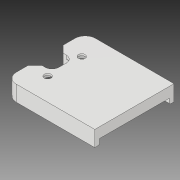
# Autodesk Inventor part: Kondensatorschutz
Saved by Autodesk Inventor 2019.4 (Build 234330000, 330)
## iProperties
Part Number: Kondensatorschutz
Material: PC/ABS-Kunststoff
Document SubType Name: Modeling
Designer: rYan
Density: 0.357273 g/cm^3
Appearance: Glatt - Weiß
Mass: 0.598763 g
Surface Area: 16.4713 cm^2
Volume: 1.67593 cm^3
Author: rYan
Autodesk Inventor part; units mm, degrees
ref_plane "YZ Plane" through (0, 0, 0) normal (1, 0, 0) x (0, 1, 0)
ref_plane "XZ Plane" through (0, 0, 0) normal (0, 1, 0) x (-1, 0, 0)
ref_plane "XY Plane" through (0, 0, 0) normal (0, 0, 1) x (1, 0, 0)
sketch "Skizze1" plane through (0, 0, 0) normal (0, 0, 1) x (1, 0, 0)
  line L0 (3, 11.6) -> (26, 11.6)
  line L1 (26, 11.6) -> (26, -11.6)
  line L2 (26, -11.6) -> (3, -11.6)
  line L3 (0, -8.6) -> (0, 8.6)
  line L4 (-5.9456, 0) -> (31.3243, 0) projected
  arc A0 (3, 11.6) -> (0, 8.6) centre (3, 8.6) ccw
  arc A1 (0, -8.6) -> (3, -11.6) centre (3, -8.6) ccw
  point P0 (0, 0)
  point P1 (0, 11.6)
  dimension "d0" = 23.2
  dimension "d1" = 26
  dimension "d2" = 3
  constraints: 8 end point, 4 point on circle, 4 tangent, 2 centre point, 2 parallel, 2 point on line, 1 equal radius, 1 horizontal, 1 midpoint, 1 perpendicular, 1 other
  measures "d0" distance of L0.end L1.end
  measures "d1" distance of point (0, 11.6) L0.end
  measures "d2" radius of A0
extrude "Extrusion1" add sketch "Skizze1" along normal blind 3
sketch "Skizze2" plane through (0, 0, 0) normal (0, 0, -1) x (-1, 0, 0)
  line L0 (0, -8.6) -> (0, 8.6) projected
  arc A0 (0, 8.6) -> (-3, 11.6) centre (-3, 8.6) ccw projected
  line L1 (-3, 11.6) -> (-26, 11.6) projected
  line L2 (-26, 11.6) -> (-26, -11.6) projected
  line L3 (-26, -11.6) -> (-3, -11.6) projected
  arc A1 (-3, -11.6) -> (0, -8.6) centre (-3, -8.6) ccw projected
  line L4 (-3, -10.2) -> (-26, -10.2)
  line L5 (-26, -10.2) -> (-26, 10.2)
  line L6 (-26, 10.2) -> (-3, 10.2)
  arc A2 (-1.4, 8.6) -> (-3, 10.2) centre (-3, 8.6) ccw
  line L7 (-1.4, 8.6) -> (-1.4, -8.6)
  arc A3 (-3, -10.2) -> (-1.4, -8.6) centre (-3, -8.6) ccw
  line L8 (0, -8.6) -> (0, 8.6) projected
  point P0 (0, 0)
  dimension "d8" = 1.4
  constraints: 8 end point, 4 point on circle, 2 centre point, 1 collinear, 1 tangent, 3 other
  measures "d8" distance between parallel lines of L3 L4
extrude "Extrusion2" add sketch "Skizze2" along normal blind 1.6 contours A1 L3 L2 L4 A3 L7 A2 L6 L1 A0 L0
sketch "Skizze3" plane through (0, 0, 3) normal (0, 0, 1) x (1, 0, 0)
  line L0 (0, 8.6) -> (0, -8.6) projected
  arc A0 (0, -8.6) -> (3, -11.6) centre (3, -8.6) ccw projected
  line L1 (3, -11.6) -> (26, -11.6) projected
  line L2 (26, -11.6) -> (26, 11.6) projected
  line L3 (26, 11.6) -> (3, 11.6) projected
  arc A1 (3, 11.6) -> (0, 8.6) centre (3, 8.6) ccw projected
  line L4 (0, 8.6) -> (0, -8.6) projected
  line L5 (0, 3.1) -> (5, 3.1)
  line L6 (5, 3.1) -> (5, -3.1)
  line L7 (5, -3.1) -> (0, -3.1)
  line L8 (0, -3.1) -> (0, 3.1)
  line L9 (-5.6971, 0) -> (31.2828, 0) projected
  point P0 (0, 0)
  dimension "d9" = 8.5
  dimension "d10" = 5
  constraints: 8 end point, 2 parallel, 1 horizontal, 1 perpendicular, 1 point on line, 1 other
  measures "d9" distance between parallel lines of L3 L5
  measures "d10" distance of L5.start L5.end
extrude "Extrusion3" cut sketch "Skizze3" against normal through all contours L5 L6 L9 L0 | L9 L6 L7 L0
sketch "Skizze5" plane through (0, 0, 0) normal (0, 0, -1) x (-1, 0, 0)
  line L0 (-5, -3.1) -> (-5, 3.1) projected
  line L1 (-31.2, 0) -> (5.2, 0) projected
  line L2 (-5, 3.1) -> (-5, -3.1) projected
  line L3 (-5, -3.1) -> (-9.4, -3.1)
  line L4 (-9.4, -3.1) -> (-9.4, 3.1)
  line L5 (-9.4, 3.1) -> (-5, 3.1)
  line L6 (-5, 3.1) -> (-5, -3.1)
  line L7 (-1.4, -8.6) -> (-1.4, -3.1) projected
  point P0 (0, 0)
  dimension "d23" = 8
  constraints: 8 end point, 2 parallel, 1 horizontal, 1 perpendicular, 1 point on line
  measures "d23" distance between parallel lines of L4 L7
extrude "Extrusion4" cut sketch "Skizze5" against normal blind 2
sketch "Skizze4" plane through (0, 0, 0) normal (0, 0, -1) x (-1, 0, 0)
  line L0 (0, -16.24) -> (0, 16.24) projected
  line L1 (-31.2, 0) -> (5.2, 0) projected
  line L2 (-1.4, -3.1) -> (-1.4, -8.6) projected
  point P0 (0, 0)
  point P1 (-5.6, -5)
  point P2 (-5.6, 5)
  dimension "d13" = 10
  dimension "d15" = 4.2
  constraints: 1 symmetric about line
  measures "d13" distance of point (-5.6, 5) point (-5.6, -5)
  measures "d15" distance from line of point (-5.6, -5) L2
hole "Bohrung1" at (5.6, -5, 0) at (5.6, 5, 0) direction (0, 0, 1) diameter 2 end through all countersink diameter 7 countersink angle 90
fillet "Rundung1" radius 2 2 edges at (5, 3.1, 2.5) (5, -3.1, 2.5)
sketch "Skizze6" plane through (0, 0, -1.6) normal (0, 0, -1) x (-1, 0, 0)
  line L0 (0, -3.1) -> (-1.4, -3.1) projected
  line L1 (-1.4, -3.1) -> (-1.4, -8.6) projected
  arc A0 (-3, -10.2) -> (-1.4, -8.6) centre (-3, -8.6) ccw projected
  line L2 (-3, -10.2) -> (-26, -10.2) projected
  line L3 (-26, -10.2) -> (-26, -11.6) projected
  line L4 (-26, -11.6) -> (-3, -11.6) projected
  arc A1 (-3, -11.6) -> (0, -8.6) centre (-3, -8.6) ccw projected
  line L5 (0, -8.6) -> (0, -3.1) projected
  line L6 (-1.4, 3.1) -> (0, 3.1) projected
  line L7 (0, 3.1) -> (0, 8.6) projected
  arc A2 (0, 8.6) -> (-3, 11.6) centre (-3, 8.6) ccw projected
  line L8 (-3, 11.6) -> (-26, 11.6) projected
  line L9 (-26, 11.6) -> (-26, 10.2) projected
  line L10 (-26, 10.2) -> (-3, 10.2) projected
  arc A3 (-1.4, 8.6) -> (-3, 10.2) centre (-3, 8.6) ccw projected
  line L11 (-1.4, 8.6) -> (-1.4, 3.1) projected
  line L12 (-3, -11.6) -> (-26, -11.6) projected
  line L13 (-26, -10.2) -> (-3, -10.2) projected
  line L14 (-26, -11.6) -> (-21, -11.6)
  line L15 (-21, -11.6) -> (-21, -10.2)
  line L16 (-21, -10.2) -> (-26, -10.2)
  line L17 (-26, -10.2) -> (-26, -11.6)
  point P0 (0, 0)
  dimension "d27" = 5
  constraints: 8 end point, 2 parallel, 1 horizontal, 1 perpendicular, 1 point on line
  measures "d27" distance between parallel lines of L3 L15
extrude "Extrusion5" [suppressed]
sketch "Skizze8" plane through (26, -11.6, 3) normal (1, 0, 0) x (0, 0, -1)
  line L0 (0, 23.2) -> (4.6, 23.2) projected
  line L1 (0, 0) -> (0, 23.2) projected
  line L2 (0, 0) -> (4.6, 0) projected
  line L3 (4.6, 1.4) -> (3, 1.4) projected
  line L4 (3, 21.8) -> (3, 1.4) projected
  line L5 (3, 21.8) -> (4.6, 21.8) projected
  line L6 (4.6, 23.2) -> (4.6, 21.8) projected
  line L7 (6.6, 1.4) -> (5.5, 2.0351)
  line L8 (5.5, 2.0351) -> (4.4, 1.4)
  line L9 (6.6, 1.4) -> (3, 1.4) projected
  line L10 (5.5, 2.0351) -> (5.5, 1.4) construction
  line L11 (6.6, 1.4) -> (4.4, 1.4)
  line L12 (4.6, 1.4) -> (4.6, 0) projected
  point P0 (3, 11.6)
  dimension "d30" = 2.2
  dimension "d34" = 30
  constraints: 8 end point, 2 point on line, 1 collinear, 1 vertical
  measures "d30" distance of L8.end L7.start
  measures "d34" angle of L3 L7
extrude "Extrusion6" [suppressed]
sketch "Skizze9" plane through (0, 0, -1.6) normal (0, 0, -1) x (-1, 0, 0)
  line L0 (-26, -11.6) -> (-3, -11.6) projected
  arc A0 (-3, -11.6) -> (0, -8.6) centre (-3, -8.6) ccw projected
  line L1 (0, -8.6) -> (0, -3.1) projected
  line L2 (0, -3.1) -> (-1.4, -3.1) projected
  line L3 (-1.4, -3.1) -> (-1.4, -8.6) projected
  arc A1 (-3, -10.2) -> (-1.4, -8.6) centre (-3, -8.6) ccw projected
  line L4 (-3, -10.2) -> (-26, -10.2) projected
  line L5 (-26, -11.6) -> (-3, -11.6) projected
  line L6 (-21, -11.6) -> (-20, -11.6)
  line L7 (-20, -11.6) -> (-20, -9.2)
  line L8 (-20, -9.2) -> (-21, -9.2)
  line L9 (-21, -10.6) -> (-21, -11.6)
  line L10 (-20, -9.2) -> (-26, -9.2)
  line L11 (-26, -9.2) -> (-26, -10.6)
  line L12 (-20, -10.2) -> (-20, -9.2)
  line L13 (-21, -10.6) -> (-26, -10.6)
  line L14 (-26, -10.2) -> (-26, -11.6) projected
  point P0 (0, 0)
  dimension "d40" = 1
  dimension "d41" = 1.4
  constraints: 16 end point, 4 parallel, 2 horizontal, 2 perpendicular, 1 point on line
  measures "d40" distance between parallel lines of L4 L10
  measures "d41" distance between parallel lines of L13 L10
extrude "Extrusion7" [suppressed]
mirror "Spiegeln1" [suppressed]
chamfer "Fase1" [suppressed]
chamfer "Fase2" distance 0.3 angle 45 6 edges at (14.5, -10.2, -1.6) (1.8686, -9.7314, -1.6) (1.4, -5.85, -1.6) (14.5, 10.2, -1.6) (1.8686, 9.7314, -1.6) (1.4, 5.85, -1.6)
chamfer "Fase3" distance 2 angle 45 2 edges at (0, 3.1, 0.7) (0, -3.1, 0.7)
